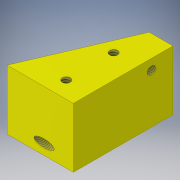
# Autodesk Inventor part: Microswitch_Bracket
Saved by Autodesk Inventor 2016 (Build 200138000, 138)
## iProperties
Created: 2016-05-07
Part Number: Microswitch_Bracket
Material: ABS Plastic
Document SubType Name: Modeling
Designer: agmle
Density: 1.06 g/cm^3
Appearance: Smooth - Yellow
Mass: 5.25736 g
Surface Area: 22.173 cm^2
Volume: 4.95977 cm^3
Author: agmle
Autodesk Inventor part; units mm, degrees
ref_plane "YZ Plane" through (0, 0, 0) normal (1, 0, 0) x (0, 1, 0)
ref_plane "XZ Plane" through (0, 0, 0) normal (0, 1, 0) x (-1, 0, 0)
ref_plane "XY Plane" through (0, 0, 0) normal (0, 0, 1) x (1, 0, 0)
sketch "Sketch1" plane through (0, 0, 0) normal (0, 1, 0) x (-1, 0, 0)
  line L0 (0, 0) -> (17.7417, 0)
  line L1 (17.7417, 0) -> (6.35, -26.6689)
  line L2 (6.35, -26.6689) -> (0, -26.6689)
  line L3 (0, -26.6689) -> (0, 0)
  dimension "d0" = 23.13
  dimension "d1" = 29
  dimension "d2" = 6.35
  constraints: 8 end point, 1 horizontal, 1 parallel, 1 perpendicular
  measures "d0" angle of L3 L1
  measures "d1" distance of L0.end L1.end
  measures "d2" distance of L1.end L2.end
extrude "Extrusion1" add sketch "Sketch1" along normal blind 16
sketch "Sketch2" plane through (-17.7417, 0, 0) normal (-0.9196159, 0, -0.3928187) x (-0.3928187, 0, 0.9196159)
  line L0 (-29, 16) -> (0, 16) construction
  line L1 (-29, 0) -> (-29, 16) construction
  line L2 (0, 0) -> (-29, 0) construction
  line L3 (0, 0) -> (0, 16) construction
  point P0 (-6.9693, 0)
  point P1 (-3.8988, 2.8114)
  point P2 (-26.2, 13.2)
  dimension "d5" = 2.8
  dimension "d6" = 2.8
  dimension "d26" = 22.3012
  dimension "d27" = 10.3886
  measures "d5" distance from line of L0 point (-26.2, 13.2)
  measures "d6" distance from line of L1 point (-26.2, 13.2)
  measures "d26" horizontal distance of point (-3.899, 2.811) point (-26.2, 13.2)
  measures "d27" vertical distance of point (-26.2, 13.2) point (-3.899, 2.811)
hole "Hole1" at (-16.2102, 2.8114, -3.5854) at (-7.4499, 13.2, -24.0939) direction (0.9196159, 0, 0.3928187) diameter 2.159 end through all
sketch "Sketch3" plane through (0, 16, 0) normal (0, 1, 0) x (1, 0, 0)
  line L0 (-17.7417, 0) -> (0, 0) construction
  line L1 (-6.35, 0) -> (-6.35, 26.6689) construction
  line L2 (0, 26.6689) -> (-6.35, 26.6689) construction
  line L3 (0, 0) -> (0, 26.6689) construction
  point P0 (-6.35, 4.445)
  point P1 (-6.35, 17.1439)
  dimension "d16" = 6.35
  dimension "d17" = 4.445
  dimension "d18" = 9.525
  dimension "d28" = 12.6989
  constraints: 4 point on line, 2 end point, 1 parallel
  measures "d16" distance between parallel lines of L3 L1
  measures "d17" distance from line of L0 point (-6.35, 4.445)
  measures "d18" distance from line of L2 point (-6.35, 17.144)
  measures "d28" distance of point (-6.35, 4.445) point (-6.35, 17.144)
hole "Hole2" at (-6.35, 16, -4.445) at (-6.35, 16, -17.1439) direction (0, -1, 0) diameter 2.159 end through all
equation "\"d6\" = d5"
body "Solid1"
